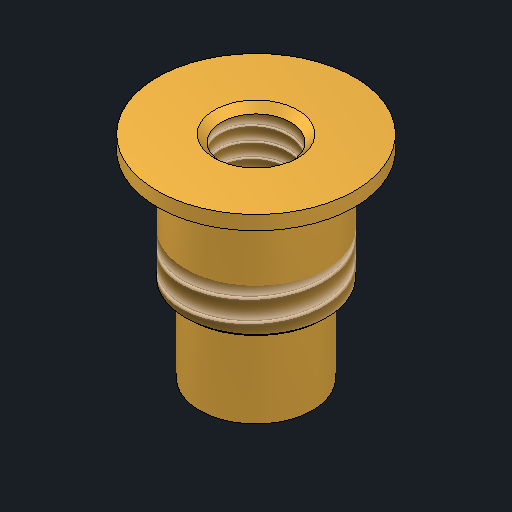
# Autodesk Inventor part: KN-00-02-02
Saved by Autodesk Inventor 2025.2 (Build 292293000, 293)
## iProperties
Created: 2025-04-12
Part Number: KN-00-02-02
Material: CuZn40
Document SubType Name: Modeling
Designer: Kacper Mik
Density: 8.47 g/cm^3
Appearance: Brass - Satin
Author: Kacper Mik
Autodesk Inventor part; units mm, degrees
ref_plane "YZ Plane" through (0, 0, 0) normal (1, 0, 0) x (0, 1, 0)
ref_plane "XZ Plane" through (0, 0, 0) normal (0, 1, 0) x (-1, 0, 0)
ref_plane "XY Plane" through (0, 0, 0) normal (0, 0, 1) x (1, 0, 0)
sketch "Sketch1" plane through (0, 0, 0) normal (0, 1, 0) x (-1, 0, 0)
  circle A0 centre (0, 0) radius 5
  dimension "d0" = 10
  constraints: 1 centre point, 1 coincident
  measures "d0" diameter of A0
extrude "Extrusion1" add sketch "Sketch1" along normal blind 8
sketch "Sketch3" plane through (0, 8, 0) normal (0, 1, 0) x (1, 0, 0)
  circle A0 centre (0, 0) radius 7
  dimension "d10" = 14
  constraints: 1 centre point
  measures "d10" diameter of A0
extrude "Extrusion2" add sketch "Sketch3" along normal blind 1
chamfer "Chamfer1" distance 0.2 angle 45 1 edges at (5, 0, 0)
sketch "Sketch4" plane through (0, 0, 0) normal (0, -1, 0) x (1, 0, 0)
  circle A0 centre (0, 0) radius 4
  dimension "d18" = 8
  constraints: 1 centre point, 1 coincident
  measures "d18" diameter of A0
extrude "Extrusion3" add sketch "Sketch4" along normal blind 6
sketch "Sketch5" plane through (0, 9, 0) normal (0, 1, 0) x (1, 0, 0)
  point P0 (0, 0)
  point P1 (0, 0)
  constraints: 1 coincident
hole "Hole2" at (0, 9, 0) direction (0, -1, 0) diameter 4.917 end through all thread size "M6x1" class "6H" standard "ISO Metric profile"
chamfer "Chamfer3" distance 0.5 angle 45 1 edges at (0, 9, -2.4585)
chamfer "Chamfer4" distance 0.5 angle 45 1 edges at (0, -6, -2.4585)
thread "Thread2" size "M10x1.5" class "6g" standard "ISO Metric profile" length 3
sketch "Sketch7" plane through (0, 0, 0) normal (0, 0, 1) x (1, 0, 0)
  line L0 (5, 8) -> (-5, 8) construction
  line L1 (-5, 0.2) -> (5, 0.2) construction
  line L2 (7, 9) -> (-7, 9) construction
  line L3 (7, 8) -> (-7, 8) construction
  line L4 (-5, 8) -> (-4.8, 8)
  line L5 (-4.8, 8) -> (-4.8, 7.8)
  line L6 (-4.8, 7.8) -> (-5, 7.8)
  line L7 (-5, 7.8) -> (-5, 8)
  line L8 (0, -9) -> (0, 12) projected
  point P0 (0, 0)
  dimension "d39" = 0.2
  dimension "d40" = 0.2
  constraints: 8 end point, 2 parallel, 1 horizontal, 1 perpendicular
  measures "d39" distance of L4.end L5.end
  measures "d40" distance of L5.end L6.end
revolve "Revolution1" cut sketch "Sketch7" angle 360 about axis through (0, -10, 0) along (0, 1, 0)
body "Solid1"
